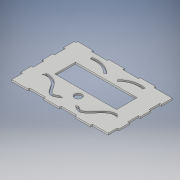
# Autodesk Inventor part: DEPAN
Saved by Autodesk Inventor 2019 (Build 230136000, 136)
## iProperties
Created: 2019-11-24
Part Number: DEPAN
Material: Generic
Document SubType Name: Modeling
Designer: User
Density: 1 g/cm^3
Appearance: Default
Author: User
Autodesk Inventor part; units mm, degrees
ref_plane "YZ Plane" through (0, 0, 0) normal (1, 0, 0) x (0, 1, 0)
ref_plane "XZ Plane" through (0, 0, 0) normal (0, 1, 0) x (-1, 0, 0)
ref_plane "XY Plane" through (0, 0, 0) normal (0, 0, 1) x (1, 0, 0)
sketch "Sketch1" plane through (0, 0, 0) normal (0, 1, 0) x (-1, 0, 0)
  line L0 (-0.0001, 6.6208) -> (-36.0001, 6.6209)
  line L1 (-36.0001, 6.6209) -> (-36.0001, -17.3791)
  line L2 (-36.0001, -17.3791) -> (-0.0001, -17.3792)
  spline S0 degree 4 poles (-44.4384, 14.3786) (-36.2284, 11.2685) (-27.2938, 14.8727) (-22.5204, 41.5888) (-8.0598, 26.2519) knots 0 0 0 0 0 1 1 1 1 1
  line L3 (-6.3049, -24.2635) -> (-8.0612, -22.4841)
  line L4 (-8.0598, 26.2519) -> (-11.3063, 25.8252)
  arc A0 (-31.0689, -31.7614) -> (-6.3049, -24.2635) centre (-25.6028, -5.1706) ccw
  arc A1 (-30.5655, -29.3126) -> (-8.0612, -22.4841) centre (-25.6028, -5.1706) ccw
  line L5 (-44.4384, 14.3786) -> (-41.1945, 11.0226)
  line L6 (-31.0689, -31.7614) -> (-30.5655, -29.3126)
  circle A2 centre (0, 15.3641) radius 4.25
  line L7 (-0.0001, 6.6208) -> (35.9999, 6.6207)
  line L8 (35.9999, 6.6207) -> (35.9999, -17.3793)
  line L9 (35.9999, -17.3793) -> (-0.0001, -17.3792)
  spline S1 degree 4 poles (43.273, 14.3755) (37.404, 11.9167) (18.0485, 12.8899) (28.5936, 42.1208) (7.1716, 26.2518) knots 0 0 0 0 0 1 1 1 1 1
  line L10 (0.0001, 27.0593) -> (0.0001, 27.2937)
  line L11 (6.2819, -24.2402) -> (8.0612, -22.4841)
  arc A3 (6.2819, -24.2402) -> (31.0689, -31.7614) centre (25.6028, -5.1706) ccw
  line L12 (31.0689, -31.7614) -> (30.5655, -29.3126)
  arc A4 (8.0612, -22.4841) -> (30.5655, -29.3126) centre (25.6028, -5.1706) ccw
  line L13 (7.1716, 26.2518) -> (10.9432, 25.8271)
  line L14 (43.273, 14.3755) -> (40.7807, 11.2249)
  line L15 (55.6, -39.5) -> (55.6, -37.5)
  line L16 (55.6, -39.5) -> (37.3, -39.5)
  line L17 (37.3, -39.5) -> (37.3, -37.5)
  line L18 (37.3, -37.5) -> (19, -37.5)
  line L19 (19, -37.5) -> (19, -39.5)
  line L20 (19, -39.5) -> (0.7, -39.5)
  line L21 (0.7, -39.5) -> (0.7, -37.5)
  line L22 (0.7, -37.5) -> (-17.6, -37.5)
  line L23 (-17.6, -37.5) -> (-17.6, -39.5)
  line L24 (-17.6, -39.5) -> (-35.9, -39.5)
  line L25 (-35.9, -39.5) -> (-35.9, -37.5)
  line L26 (-35.9, -37.5) -> (-55, -37.5)
  line L27 (-55, -37.5) -> (-57, -37.5)
  line L28 (-57, -37.5) -> (-57, -25)
  line L29 (-57, -25) -> (-55, -25)
  line L30 (-55, -25) -> (-55, -12.5)
  line L31 (-55, -12.5) -> (-57, -12.5)
  line L32 (-57, -12.5) -> (-57, 0)
  line L33 (-57, 0) -> (-55, 0)
  line L34 (-55, 0) -> (-55, 12.5)
  line L35 (-55, 12.5) -> (-57, 12.5)
  line L36 (-57, 12.5) -> (-57, 25)
  line L37 (-57, 25) -> (-55, 25)
  line L38 (-55, 25) -> (-55, 35.5)
  line L39 (-35.9999, 39.5001) -> (-35.9, 39.5001)
  line L40 (55.6, 37.5) -> (55.6, 25)
  line L41 (55.6, 25) -> (57.6, 25)
  line L42 (57.6, 25) -> (57.6, 12.5)
  line L43 (57.6, 12.5) -> (55.6, 12.5)
  line L44 (55.6, 12.5) -> (55.6, 0)
  line L45 (55.6, 0) -> (57.6, 0)
  line L46 (57.6, 0) -> (57.6, -12.5)
  line L47 (57.6, -12.5) -> (55.6, -12.5)
  line L48 (55.6, -12.5) -> (55.6, -25)
  line L49 (55.6, -25) -> (57.6, -25)
  line L50 (57.6, -25) -> (57.6, -37.5)
  line L51 (57.6, -37.5) -> (55.6, -37.5)
  line L52 (-55, 35.5) -> (-36.7, 35.5)
  line L53 (-36.7, 35.5) -> (-36.7, 37.5)
  line L54 (-18.4, 37.5) -> (-36.7, 37.5)
  line L55 (-18.4, 37.5) -> (-18.4, 35.5)
  line L56 (-18.4, 35.5) -> (-0.1, 35.5)
  line L57 (-0.1, 35.5) -> (-0.1, 37.5)
  line L58 (-0.1, 37.5) -> (18.2, 37.5)
  line L59 (18.2, 37.5) -> (18.2, 35.5)
  line L60 (18.2, 35.5) -> (36.5, 35.5)
  line L61 (36.5, 35.5) -> (36.5, 37.5)
  line L62 (36.5, 37.5) -> (55.6, 37.5)
  line L63 (-0.0999, 39.5) -> (0.0003, 39.5)
  spline S2 degree 5 poles (-41.1945, 11.0226) (-40.5347, 10.9757) (-39.8718, 10.9722) (-39.2095, 11.0146) (-37.7702, 11.2089) (-36.3743, 11.6152) (-35.635, 11.8954) (-34.1715, 12.5731) (-32.8071, 13.4338) (-32.1369, 13.9122) (-30.8093, 14.9581) (-29.5704, 16.1077) (-28.9543, 16.7178) (-27.7354, 17.9857) (-26.5633, 19.2972) (-25.9765, 19.9688) (-24.8295, 21.2939) (-23.6753, 22.6125) (-23.1021, 23.2546) (-22.013, 24.4315) (-20.8566, 25.5431) (-20.3018, 26.0367) (-19.2854, 26.8522) (-18.16, 27.5031) (-17.6548, 27.743) (-16.5977, 28.0884) (-15.483, 28.0865) (-14.9396, 27.9807) (-13.8172, 27.608) (-12.7985, 27.0033) (-12.2788, 26.6377) (-11.7827, 26.2428) (-11.3064, 25.8252) knots 0 0 0 0 0 0 0.089804 0.089804 0.089804 0.196736 0.196736 0.196736 0.308348 0.308348 0.308348 0.426015 0.426015 0.426015 0.547114 0.547114 0.547114 0.663954 0.663954 0.663954 0.764764 0.764764 0.764764 0.840174 0.840174 0.840174 0.913976 0.913976 0.913976 1 1 1 1 1 1
  spline S3 degree 5 poles (40.7807, 11.2249) (40.1484, 11.1565) (39.5125, 11.1211) (38.8755, 11.1172) (37.4673, 11.1777) (36.073, 11.3895) (35.3163, 11.5507) (33.797, 11.9702) (32.3389, 12.5693) (31.6157, 12.9197) (30.2022, 13.7122) (28.8891, 14.6623) (28.2541, 15.1779) (27.0405, 16.2716) (25.9335, 17.473) (25.4056, 18.0958) (24.4144, 19.3527) (23.4953, 20.6632) (23.0584, 21.3149) (22.2516, 22.555) (21.4527, 23.8001) (21.0736, 24.3826) (20.3954, 25.3906) (19.6462, 26.3476) (19.308, 26.7414) (18.6927, 27.3676) (17.9562, 27.838) (17.6323, 27.9896) (16.706, 28.2187) (15.7507, 28.0855) (15.1792, 27.9365) (13.9448, 27.5092) (12.7769, 26.9259) (12.1537, 26.5791) (11.5431, 26.2114) (10.9432, 25.8271) knots 0 0 0 0 0 0 0.084867 0.084867 0.084867 0.187859 0.187859 0.187859 0.29482 0.29482 0.29482 0.403756 0.403756 0.403756 0.512584 0.512584 0.512584 0.617265 0.617265 0.617265 0.709997 0.709997 0.709997 0.7793 0.7793 0.7793 0.826133 0.826133 0.826133 0.904929 0.904929 0.904929 1 1 1 1 1 1
  point P0 (0, 0)
  point P1 (0, 0)
  point P2 (-37.8426, 13.8908)
  point P3 (-30.3235, 19.0112)
  point P4 (-20.7788, 28.8828)
  point P5 (36.4928, 13.8824)
  point P6 (27.9279, 19.022)
  point P7 (21.2262, 28.3156)
  point P8 (-55, 37.5)
  point P9 (18.2001, 39.5)
  dimension "d0" = 55.6
  dimension "d1" = 39.5
  dimension "d2" = 2
  dimension "d3" = 18.3
  dimension "d4" = 18.3
  dimension "d5" = 2
  dimension "d6" = 18.3
  dimension "d7" = 18.3
  dimension "d8" = 18.3
  dimension "d9" = 2
  dimension "d10" = 19.1
  dimension "d11" = 2
  dimension "d12" = 12.5
  dimension "d13" = 12.5
  dimension "d14" = 2
  dimension "d15" = 12.5
  dimension "d16" = 12.5
  dimension "d17" = 2
  dimension "d18" = 12.5
  dimension "d33" = 2
  dimension "d34" = 12.5
  dimension "d35" = 2
  dimension "d36" = 12.5
  dimension "d37" = 2
  dimension "d38" = 12.5
  dimension "d39" = 2
  dimension "d40" = 12.5
  dimension "d41" = 12.5
  constraints: 128 end point, 32 point on line, 19 perpendicular, 8 point on circle, 5 centre point, 4 vertical, 3 horizontal, 1 parallel, 18 other
  measures "d0" horizontal distance of point (0, 0) L15.start
  measures "d1" vertical distance of point (0, 0) L15.start
  measures "d2" distance of L15.start L15.end
  measures "d3" distance of L15.start L16.end
  measures "d4" distance of L17.end L18.end
  measures "d5" distance of L18.end L19.end
  measures "d6" distance of L19.end L20.end
  measures "d7" distance of L21.end L22.end
  measures "d8" distance of L23.end L24.end
  measures "d9" distance of L24.end L25.end
  measures "d10" distance of L25.end L26.end
  measures "d11" distance of L26.end L27.end
  measures "d12" distance of L27.end L28.end
  measures "d13" distance of L29.end L30.end
  measures "d14" distance of L30.end L31.end
  measures "d15" distance of L31.end L32.end
  measures "d16" distance of L33.end L34.end
  measures "d17" distance of L34.end L35.end
  measures "d18" distance of L35.end L36.end
  measures "d33" distance of L40.end L41.end
  measures "d34" distance of L41.end L42.end
  measures "d35" distance of L42.end L43.end
  measures "d36" distance of L43.end L44.end
  measures "d37" distance of L44.end L45.end
  measures "d38" distance of L45.end L46.end
  measures "d39" distance of L46.end L47.end
  measures "d40" distance of L47.end L48.end
  measures "d41" distance of L49.end L50.end
extrude "Extrusion1" add sketch "Sketch1" along normal blind 2
body "Solid1"
